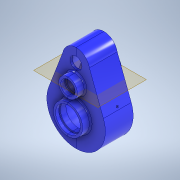
# Autodesk Inventor part: Корпус
Saved by Autodesk Inventor 2021 (Build 250183000, 183)
## iProperties
Created: 2023-03-11
Part Number: Корпус
Material: Сталь
Document SubType Name: Modeling
Designer: gdevc
Density: 7.85 g/cm^3
Appearance: Синий — малярная краска — глянцевая
Author: gdevc
Autodesk Inventor part; units mm, degrees
ref_plane "YZ Plane" through (0, 0, 0) normal (1, 0, 0) x (0, 1, 0)
ref_plane "XY Plane" through (0, 0, 0) normal (0, 0, 1) x (1, 0, 0)
sketch "Эскиз1" plane through (0, 0, 0) normal (0, 0, 1) x (1, 0, 0)
  line L0 (-40.4297, 169.8146) -> (-91.8672, 35.0692)
  arc A0 (-91.8672, 35.0692) -> (95.7766, 22.277) centre (0, 0) ccw
  arc A1 (40.4297, 169.8146) -> (-40.4297, 169.8146) centre (0, 163) ccw
  line L1 (-40.4297, 169.8146) -> (-91.8672, 35.0692)
  arc A2 (-91.8672, 35.0692) -> (95.7766, 22.277) centre (0, 0) ccw
  arc A3 (40.4297, 169.8146) -> (-40.4297, 169.8146) centre (0, 163) ccw
  line L2 (-40.4297, 169.8146) -> (-91.8672, 35.0692)
  arc A4 (-91.8672, 35.0692) -> (95.7766, 22.277) centre (0, 0) ccw
  arc A5 (40.4297, 169.8146) -> (-40.4297, 169.8146) centre (0, 163) ccw
  arc A6 (-91.8672, 35.0692) -> (91.8672, 35.0692) centre (0, 0) ccw
  arc A7 (40.4297, 169.8146) -> (-40.4297, 169.8146) centre (0, 163) ccw
  line L3 (-40.4297, 169.8146) -> (-91.8672, 35.0692)
  line L4 (40.4297, 169.8146) -> (91.8672, 35.0692)
  line L5 (-40.4297, 169.8146) -> (-91.8672, 35.0692)
  arc A8 (-91.8672, 35.0692) -> (91.8672, 35.0692) centre (0, 0) ccw
  arc A9 (40.4297, 169.8146) -> (-40.4297, 169.8146) centre (0, 163) ccw
  line L6 (40.4297, 169.8146) -> (91.8672, 35.0692)
  arc A10 (48.3184, 171.1443) -> (-48.3184, 171.1443) centre (0, 163) ccw
  line L7 (-47.9037, 172.6677) -> (-99.3411, 37.9223)
  arc A11 (-99.3411, 37.9223) -> (103.5686, 24.0893) centre (0, 0) ccw
  line L8 (47.9037, 172.6677) -> (99.3411, 37.9223)
  arc A12 (-99.3411, 37.9223) -> (99.3411, 37.9223) centre (0, 0) ccw
  point P0 (103.5686, 24.0893)
  point P1 (99.3411, 37.9223)
  point P2 (48.1739, 171.9598)
  point P3 (-48.1739, 171.9598)
  point P4 (95.7766, 22.277)
  dimension "d0" = 8
  dimension "d1" = 8
  dimension "d2" = 8
  dimension "d3" = 8
  dimension "d4" = 8
  constraints: 26 point on circle, 18 end point, 13 centre point, 2 parallel
  measures "d0" radial gap between concentric circles of A1 A10
  measures "d1" distance between parallel lines of L0 L7
  measures "d2" radial gap between concentric circles of A0 A11
  measures "d3" distance between parallel lines of L4 L8
  measures "d4" radial gap between concentric circles of A6 A12
extrude "Выдавливание1" add sketch "Эскиз1" along normal mid plane 101
sketch "Эскиз2" plane through (0, 0, 50.5) normal (0, 0, 1) x (1, 0, 0)
  arc A0 (40.4297, 169.8146) -> (-40.4297, 169.8146) centre (0, 163) ccw projected
  line L0 (-91.8672, 35.0692) -> (-40.4297, 169.8146) projected
  line L1 (40.4297, 169.8146) -> (91.8672, 35.0692) projected
  arc A1 (-91.8672, 35.0692) -> (91.8672, 35.0692) centre (0, 0) ccw projected
extrude "Крышка правая" add sketch "Эскиз2" against normal blind 8
sketch "Эскиз3" plane through (0, 0, -50.5) normal (0, 0, -1) x (-1, 0, 0)
  arc A0 (40.4297, 169.8146) -> (-40.4297, 169.8146) centre (0, 163) ccw projected
  line L0 (-91.8672, 35.0692) -> (-40.4297, 169.8146) projected
  arc A1 (-91.8672, 35.0692) -> (91.8672, 35.0692) centre (0, 0) ccw projected
  line L1 (40.4297, 169.8146) -> (91.8672, 35.0692) projected
  arc A2 (40.4297, 169.8146) -> (-40.4297, 169.8146) centre (0, 163) ccw projected
  point P0 (-40.4297, 169.8146)
  point P1 (40.4297, 169.8146)
extrude "Крышка левая" add sketch "Эскиз3" against normal blind 8
sketch "Эскиз4" plane through (0, 0, 50.5) normal (0, 0, 1) x (1, 0, 0)
  circle A0 centre (0, 163) radius 21.5
  point P0 (0, 0)
  dimension "d11" = 43
  constraints: 1 centre point, 1 coincident
  measures "d11" diameter of A0
extrude "Под валл" cut sketch "Эскиз4" against normal blind 8
sketch "Эскиз5" plane through (0, 0, -50.5) normal (0, 0, -1) x (-1, 0, 0)
  circle A0 centre (0, 0) radius 45
  dimension "d15" = 90
  constraints: 1 centre point, 1 coincident
  measures "d15" diameter of A0
extrude "Под валл тих" cut sketch "Эскиз5" against normal blind 37
sketch "Эскиз7" plane through (0, 0, -50.5) normal (0, 0, -1) x (-1, 0, 0)
  circle A0 centre (0, 0) radius 45 projected
  circle A1 centre (0, 0) radius 53
  dimension "d19" = 8
  constraints: 1 centre point
  measures "d19" radial gap between concentric circles of A0 A1
extrude "Выдавливание6" add sketch "Эскиз7" along normal blind 29.5
sketch "Эскиз9" plane through (0, 0, 50.5) normal (0, 0, 1) x (1, 0, 0)
  circle A0 centre (0, 0) radius 53 projected
  arc A1 (0, 45) -> (0, -45) centre (0, 0) ccw projected
  arc A2 (0, -45) -> (0, 45) centre (0, 0) ccw projected
extrude "Выдавливание11" cut sketch "Эскиз9" against normal blind 24 contours A2 A1
extrude "Выдавливание12" add sketch "Эскиз9" along normal blind 29.5
sketch "Эскиз10" plane through (0, 0, 50.5) normal (0, 0, 1) x (1, 0, 0)
  circle A0 centre (0, 100) radius 26
  point P0 (0, 0)
  dimension "d34" = 100
  dimension "d35" = 52
  constraints: 1 centre point
  measures "d34" distance of A0.centre point (0, 0)
  measures "d35" diameter of A0
extrude "Выдавливание13" cut sketch "Эскиз10" against normal through all
sketch "Эскиз11" plane through (0, 0, 50.5) normal (0, 0, 1) x (1, 0, 0)
  circle A0 centre (0, 100) radius 26 projected
  circle A1 centre (0, 100) radius 34
  point P0 (0, 0)
  dimension "d38" = 8
  constraints: 1 centre point
  measures "d38" radial gap between concentric circles of A0 A1
extrude "Выдавливание14" add sketch "Эскиз11" along normal blind 29.5
sketch "Эскиз12" plane through (0, 0, -50.5) normal (0, 0, -1) x (-1, 0, 0)
  circle A0 centre (0, 100) radius 34 projected
  circle A1 centre (0, 100) radius 26 projected
  point P0 (0, 0)
extrude "Выдавливание15" add sketch "Эскиз12" along normal blind 29.5
split body "Разделение2" result two bodies by plane through (0, 0, 0) normal (1, 0, 0) first body at (95.1804, -46.2747, 16.8333)
fillet "Сопряжение3" radius 5 6 edges at (-37.4767, -37.4767, -50.5) (-37.4767, 37.4767, -50.5) (-24.0416, 124.0416, -50.5) (-24.0416, 75.9584, -50.5) (-34, 100, 50.5) (-53, 0, 50.5)
fillet "Сопряжение4" radius 5 4 edges at (37.4767, -37.4767, 50.5) (37.4767, 37.4767, 50.5) (24.0416, 75.9584, 50.5) (24.0416, 124.0416, 50.5)
fillet "Сопряжение5" radius 5 2 edges at (34, 100, -50.5) (53, 0, -50.5)
sketch "Эскиз13" plane through (0, 0, 0) normal (0, 1, 0) x (-1, 0, 0)
  line L0 (0, -42.5) -> (0, -80) projected
  line L1 (0, -62.5) -> (-50, -62.5)
  line L2 (-50, -62.5) -> (-50, -68.5)
  line L3 (-50, -68.5) -> (0, -68.5)
  line L4 (-45, -42.5) -> (0, -42.5) projected
  line L5 (0, -62.5) -> (0, -68.5)
  line L6 (0, 0) -> (-27.5004, 0)
  line L7 (0, 62.5) -> (-50, 62.5)
  line L8 (-50, 62.5) -> (-50, 68.5)
  line L9 (-50, 68.5) -> (0, 68.5)
  line L10 (0, 62.5) -> (0, 68.5)
  line L11 (0, 80) -> (0, 42.5) projected
  dimension "d46" = 20
  dimension "d47" = 6
  dimension "d48" = 50
  constraints: 18 end point, 4 symmetric about line, 3 perpendicular, 2 point on line, 1 collinear, 1 horizontal, 1 vertical
  measures "d46" distance between parallel lines of L1 L4
  measures "d47" distance of L1.end L2.end
  measures "d48" distance between parallel lines of L2 L0
revolve "Вращение1" cut sketch "Эскиз13" angle 360 about axis through (0, 0, -42.5) along (0, 0, -1) bodies 3 2
ref_plane "РабПлоскость1" through (26, 100, 80) normal (0, 1, 0) x (-1, 0, 0)
sketch "Эскиз15" plane through (26, 100, 80) normal (0, 1, 0) x (-1, 0, 0)
  line L0 (26, -80) -> (-42.8903, -80)
  line L1 (26, -37.5) -> (26, -17.5) projected
  line L2 (26, -22.5) -> (58.5, -22.5)
  line L3 (52, 0) -> (52, -37.5) projected
  line L4 (58.5, -22.5) -> (58.5, -13.5)
  line L5 (76, -11.5) -> (26, -11.5) projected
  line L6 (58.5, -13.5) -> (26, -13.5)
  line L7 (26, 0) -> (26, -37.5) projected
  line L8 (26, 0) -> (52, 0) projected
  line L9 (26, -137.5) -> (58.5, -137.5)
  line L10 (58.5, -137.5) -> (58.5, -146.5)
  line L11 (58.5, -146.5) -> (26, -146.5)
  line L12 (26, -160) -> (26, -122.5)
  point P0 (52, -22.5)
  point P1 (52, -13.5)
  dimension "d50" = 13.5
  dimension "d51" = 9
  dimension "d52" = 65
  constraints: 16 end point, 6 symmetric about line, 3 perpendicular, 3 point on line, 1 horizontal
  measures "d50" distance between parallel lines of L8 L6
  measures "d51" distance of L2.end L4.end
  measures "d52" diameter of L4 L7
revolve "Вращение2" cut sketch "Эскиз15" angle 360 about axis through (0, 100, -80) along (0, 0, 1) bodies 2 3 contours L1 L7 L6 L3 L2 | L9 L10 L11 L12
sketch "Эскиз16" plane through (26, 100, 80) normal (0, 1, 0) x (-1, 0, 0)
  line L0 (26, -22.5) -> (58.5, -22.5)
  line L1 (58.5, -22.5) -> (58.5, -13.5)
  line L2 (58.5, -13.5) -> (26, -13.5)
  line L3 (26, -137.5) -> (52, -137.5) projected
  line L4 (26, 0) -> (26, -37.5) projected
  point P0 (26, -80)
  dimension "d54" = 9
  dimension "d55" = 57.5
  dimension "d56" = 32.5
  constraints: 6 end point, 1 horizontal, 1 perpendicular, 1 vertical
  measures "d54" distance of L0.end L1.end
  measures "d55" distance from line of point (26, -80) L0
  measures "d56" distance between parallel lines of L4 L1
revolve "Вращение3" cut sketch "Эскиз16" angle 360 about axis through (0, 100, 80) along (0, 0, -1) bodies 2 3
